Autodesk Inventor part; units mm, degrees
(part 2 of 2)
  line L870 (14, 45.5733) -> (13.8947, 45.8276) construction
  line L871 (13.8947, 45.8276) -> (13.7072, 46.0152) construction
  spline S21 degree 3 poles (13.7072, 46.0152) (13.707012, 46.015387) (13.5196, 46.2027) (13.2653, 46.308) (13, 46.308) knots 0.5 0.5 0.5 0.5 0.50000001 1 1 1 1
  line L872 (13.7072, 46.0152) -> (13.7072, 46.0152) construction
  line L873 (13.7072, 46.0152) -> (13.5196, 46.2027) construction
  line L874 (13.5196, 46.2027) -> (13.2653, 46.308) construction
  line L875 (13.2653, 46.308) -> (13, 46.308) construction
  line L876 (13, 46.308) -> (11, 46.308)
  spline S22 degree 3 poles (11, 46.308) (10.7348, 46.308) (10.4805, 46.2027) (10.2929, 46.0152) knots 0 0 0 0 0.5 0.5 0.5 0.5
  line L877 (11, 46.308) -> (10.7348, 46.308) construction
  line L878 (10.7348, 46.308) -> (10.4805, 46.2027) construction
  line L879 (10.4805, 46.2027) -> (10.2929, 46.0152) construction
  spline S23 degree 3 poles (10.2929, 46.0152) (10.292713, 46.015012) (10.1054, 45.8276) (10, 45.5733) (10, 45.308) knots 0.5 0.5 0.5 0.5 0.50000001 1 1 1 1
  line L880 (10.2929, 46.0152) -> (10.2929, 46.0152) construction
  line L881 (10.2929, 46.0152) -> (10.1054, 45.8276) construction
  line L882 (10.1054, 45.8276) -> (10, 45.5733) construction
  line L883 (10, 45.5733) -> (10, 45.308) construction
  line L884 (10, 45.308) -> (10, 41.3081)
  line L885 (10, 41.3081) -> (9, 41.3081)
  line L886 (9, 41.3081) -> (9, 39.3081)
  line L887 (7, 39.3081) -> (7, 41.3081)
  line L888 (7, 41.3081) -> (6, 41.3081)
  line L889 (6, 41.3081) -> (6, 45.308)
  spline S24 degree 3 poles (6, 45.308) (6, 45.5733) (5.8947, 45.8276) (5.7072, 46.0152) knots 0 0 0 0 0.5 0.5 0.5 0.5
  line L890 (6, 45.308) -> (6, 45.5733) construction
  line L891 (6, 45.5733) -> (5.8947, 45.8276) construction
  line L892 (5.8947, 45.8276) -> (5.7072, 46.0152) construction
  spline S25 degree 3 poles (5.7072, 46.0152) (5.707012, 46.015387) (5.5196, 46.2027) (5.2653, 46.308) (5, 46.308) knots 0.5 0.5 0.5 0.5 0.50000001 1 1 1 1
  line L893 (5.7072, 46.0152) -> (5.7072, 46.0152) construction
  line L894 (5.7072, 46.0152) -> (5.5196, 46.2027) construction
  line L895 (5.5196, 46.2027) -> (5.2653, 46.308) construction
  line L896 (5.2653, 46.308) -> (5, 46.308) construction
  line L897 (5, 46.308) -> (3, 46.308)
  spline S26 degree 3 poles (3, 46.308) (2.7348, 46.308) (2.4805, 46.2027) (2.2929, 46.0152) knots 0 0 0 0 0.5 0.5 0.5 0.5
  line L898 (3, 46.308) -> (2.7348, 46.308) construction
  line L899 (2.7348, 46.308) -> (2.4805, 46.2027) construction
  line L900 (2.4805, 46.2027) -> (2.2929, 46.0152) construction
  spline S27 degree 3 poles (2.2929, 46.0152) (2.292713, 46.015012) (2.1054, 45.8276) (2, 45.5733) (2, 45.308) knots 0.5 0.5 0.5 0.5 0.50000001 1 1 1 1
  line L901 (2.2929, 46.0152) -> (2.2929, 46.0152) construction
  line L902 (2.2929, 46.0152) -> (2.1054, 45.8276) construction
  line L903 (2.1054, 45.8276) -> (2, 45.5733) construction
  line L904 (2, 45.5733) -> (2, 45.308) construction
  line L905 (2, 45.308) -> (2, 41.3081)
  line L906 (2, 41.3081) -> (1, 41.3081)
  line L907 (1, 41.3081) -> (1, 37.6081)
  line L908 (1, 37.6081) -> (7, 37.6081)
  line L909 (7, 37.6081) -> (7, 39.0081)
  line L910 (7, 39.0081) -> (9, 39.0081)
  line L911 (9, 39.3081) -> (7, 39.3081)
  line L912 (61.6606, 20.3061) -> (65.6606, 20.3061)
  line L913 (65.6606, 20.3061) -> (65.6606, 23.3061)
  line L914 (65.6606, 23.3061) -> (61.6606, 23.3061)
  line L915 (61.6606, 23.3061) -> (61.6606, 20.3061)
  line L916 (7.1396, 50.4111) -> (11.1396, 50.4111)
  line L917 (11.1396, 50.4111) -> (11.1396, 53.4111)
  line L918 (11.1396, 53.4111) -> (7.1396, 53.4111)
  line L919 (7.1396, 53.4111) -> (7.1396, 50.4111)
  line L920 (7.1396, 57.4111) -> (11.1396, 57.4111)
  line L921 (11.1396, 57.4111) -> (11.1396, 60.4111)
  line L922 (11.1396, 60.4111) -> (7.1396, 60.4111)
  line L923 (7.1396, 60.4111) -> (7.1396, 57.4111)
  line L924 (173.9998, 64.6598) -> (168.9998, 64.6598)
  line L925 (168.9998, 64.6598) -> (168.9998, 67.6598)
  line L926 (168.9998, 67.6598) -> (173.9998, 67.6598)
  line L927 (173.9998, 67.6598) -> (173.9998, 64.6598)
  line L928 (173.9998, 5.9564) -> (168.9998, 5.9564)
  line L929 (168.9998, 5.9564) -> (168.9998, 2.9564)
  line L930 (168.9998, 2.9564) -> (173.9998, 2.9564)
  line L931 (173.9998, 2.9564) -> (173.9998, 5.9564)
  line L932 (7.1836, 64.6598) -> (12.1836, 64.6598)
  line L933 (12.1836, 64.6598) -> (12.1836, 67.6598)
  line L934 (12.1836, 67.6598) -> (7.1836, 67.6598)
  line L935 (7.1836, 67.6598) -> (7.1836, 64.6598)
  spline S28 degree 3 poles (16.2657, 59.4698) (16.2657, 60.2982) (15.5941, 60.9698) (14.7657, 60.9698) knots 0 0 0 0 1 1 1 1
  line L936 (16.2657, 59.4698) -> (16.2657, 60.2982) construction
  line L937 (16.2657, 60.2982) -> (15.5941, 60.9698) construction
  line L938 (15.5941, 60.9698) -> (14.7657, 60.9698) construction
  line L939 (14.7657, 60.9698) -> (14.7657, 60.9698) construction
  line L940 (14.7657, 60.9698) -> (13.9372, 60.9698) construction
  line L941 (13.9372, 60.9698) -> (13.2657, 60.2982) construction
  line L942 (13.2657, 60.2982) -> (13.2657, 59.4698) construction
  line L943 (13.2657, 59.4698) -> (13.2657, 59.4698) construction
  line L944 (13.2657, 59.4698) -> (13.2657, 58.6414) construction
  line L945 (13.2657, 58.6414) -> (13.9372, 57.9698) construction
  line L946 (13.9372, 57.9698) -> (14.7657, 57.9698) construction
  line L947 (14.7657, 57.9698) -> (14.7657, 57.9698) construction
  line L948 (14.7657, 57.9698) -> (15.5941, 57.9698) construction
  line L949 (15.5941, 57.9698) -> (16.2657, 58.6414) construction
  line L950 (16.2657, 58.6414) -> (16.2657, 59.4698) construction
  spline S29 degree 3 poles (16.2657, 11.2099) (16.2657, 12.0383) (15.5941, 12.7099) (14.7657, 12.7099) knots 0 0 0 0 1 1 1 1
  line L951 (16.2657, 11.2099) -> (16.2657, 12.0383) construction
  line L952 (16.2657, 12.0383) -> (15.5941, 12.7099) construction
  line L953 (15.5941, 12.7099) -> (14.7657, 12.7099) construction
  line L954 (14.7657, 12.7099) -> (14.7657, 12.7099) construction
  line L955 (14.7657, 12.7099) -> (13.9372, 12.7099) construction
  line L956 (13.9372, 12.7099) -> (13.2657, 12.0383) construction
  line L957 (13.2657, 12.0383) -> (13.2657, 11.2099) construction
  line L958 (13.2657, 11.2099) -> (13.2657, 11.2099) construction
  line L959 (13.2657, 11.2099) -> (13.2657, 10.3815) construction
  line L960 (13.2657, 10.3815) -> (13.9372, 9.7099) construction
  line L961 (13.9372, 9.7099) -> (14.7657, 9.7099) construction
  line L962 (14.7657, 9.7099) -> (14.7657, 9.7099) construction
  line L963 (14.7657, 9.7099) -> (15.5941, 9.7099) construction
  line L964 (15.5941, 9.7099) -> (16.2657, 10.3815) construction
  line L965 (16.2657, 10.3815) -> (16.2657, 11.2099) construction
  spline S30 degree 3 poles (82.3057, 14.3849) (82.3057, 15.2133) (81.6341, 15.8849) (80.8057, 15.8849) knots 0 0 0 0 1 1 1 1
  line L966 (82.3057, 14.3849) -> (82.3057, 15.2133) construction
  line L967 (82.3057, 15.2133) -> (81.6341, 15.8849) construction
  line L968 (81.6341, 15.8849) -> (80.8057, 15.8849) construction
  line L969 (80.8057, 15.8849) -> (80.8057, 15.8849) construction
  line L970 (80.8057, 15.8849) -> (79.9772, 15.8849) construction
  line L971 (79.9772, 15.8849) -> (79.3057, 15.2133) construction
  line L972 (79.3057, 15.2133) -> (79.3057, 14.3849) construction
  line L973 (79.3057, 14.3849) -> (79.3057, 14.3849) construction
  line L974 (79.3057, 14.3849) -> (79.3057, 13.5565) construction
  line L975 (79.3057, 13.5565) -> (79.9772, 12.8849) construction
  line L976 (79.9772, 12.8849) -> (80.8057, 12.8849) construction
  line L977 (80.8057, 12.8849) -> (80.8057, 12.8849) construction
  line L978 (80.8057, 12.8849) -> (81.6341, 12.8849) construction
  line L979 (81.6341, 12.8849) -> (82.3057, 13.5565) construction
  line L980 (82.3057, 13.5565) -> (82.3057, 14.3849) construction
  line L981 (0, 13.7411) -> (0, 2.9565)
  line L982 (0, 2.9564) -> (0.0018, 2.854)
  line L983 (0.0018, 2.854) -> (0.007, 2.7517)
  line L984 (0.007, 2.7517) -> (0.0158, 2.6496)
  line L985 (0.0158, 2.6496) -> (0.028, 2.5479)
  line L986 (0.028, 2.5479) -> (0.0437, 2.4467)
  line L987 (0.0437, 2.4467) -> (0.0628, 2.346)
  line L988 (0.0628, 2.346) -> (0.0853, 2.2461)
  line L989 (0.0853, 2.2461) -> (0.1113, 2.147)
  line L990 (0.1113, 2.147) -> (0.1406, 2.0489)
  line L991 (0.1406, 2.0489) -> (0.1733, 1.9518)
  line L992 (0.1733, 1.9518) -> (0.2092, 1.8558)
  line L993 (0.2092, 1.8558) -> (0.2484, 1.7612)
  line L994 (0.2484, 1.7612) -> (0.2908, 1.6679)
  line L995 (0.2908, 1.6679) -> (0.3364, 1.5762)
  line L996 (0.3364, 1.5762) -> (0.3851, 1.4861)
  line L997 (0.3851, 1.4861) -> (0.4368, 1.3976)
  line L998 (0.4368, 1.3976) -> (0.4915, 1.311)
  line L999 (0.4915, 1.311) -> (0.5491, 1.2264)
  line L1000 (0.5491, 1.2264) -> (0.6096, 1.1437)
  line L1001 (0.6096, 1.1437) -> (0.6729, 1.0631)
  line L1002 (0.6729, 1.0631) -> (0.7389, 0.9848)
  line L1003 (0.7389, 0.9848) -> (0.8075, 0.9087)
  line L1004 (0.8075, 0.9087) -> (0.8787, 0.8351)
  line L1005 (0.8787, 0.8351) -> (0.9524, 0.7639)
  line L1006 (0.9524, 0.7639) -> (1.0284, 0.6953)
  line L1007 (1.0284, 0.6953) -> (1.1068, 0.6293)
  line L1008 (1.1068, 0.6293) -> (1.1873, 0.566)
  line L1009 (1.1873, 0.566) -> (1.27, 0.5055)
  line L1010 (1.27, 0.5055) -> (1.3547, 0.4479)
  line L1011 (1.3547, 0.4479) -> (1.4413, 0.3931)
  line L1012 (1.4413, 0.3931) -> (1.5297, 0.3414)
  line L1013 (1.5297, 0.3414) -> (1.6199, 0.2927)
  line L1014 (1.6199, 0.2927) -> (1.7116, 0.2472)
  line L1015 (1.7116, 0.2472) -> (1.8048, 0.2048)
  line L1016 (1.8048, 0.2048) -> (1.8995, 0.1656)
  line L1017 (1.8995, 0.1656) -> (1.9954, 0.1296)
  line L1018 (1.9954, 0.1296) -> (2.0925, 0.097)
  line L1019 (2.0925, 0.097) -> (2.1907, 0.0676)
  line L1020 (2.1907, 0.0676) -> (2.2898, 0.0417)
  line L1021 (2.2898, 0.0417) -> (2.3897, 0.0191)
  line L1022 (2.3897, 0.0191) -> (2.4903, 0)
  line L1023 (2.4903, 0) -> (2.5916, -0.0157)
  line L1024 (2.5916, -0.0157) -> (2.6933, -0.0279)
  line L1025 (2.6933, -0.0279) -> (2.7953, -0.0366)
  line L1026 (2.7953, -0.0366) -> (2.8976, -0.0419)
  line L1027 (2.8976, -0.0419) -> (3, -0.0436)
  line L1028 (3, -0.0436) -> (84, -0.0436)
  line L1029 (84, -0.0436) -> (84.1025, -0.0419)
  line L1030 (84.1025, -0.0419) -> (84.2048, -0.0366)
  line L1031 (84.2048, -0.0366) -> (84.3068, -0.0279)
  line L1032 (84.3068, -0.0279) -> (84.4085, -0.0157)
  line L1033 (84.4085, -0.0157) -> (84.5098, 0)
  line L1034 (84.5098, 0) -> (84.6104, 0.0191)
  line L1035 (84.6104, 0.0191) -> (84.7103, 0.0417)
  line L1036 (84.7103, 0.0417) -> (84.8094, 0.0676)
  line L1037 (84.8094, 0.0676) -> (84.9076, 0.097)
  line L1038 (84.9076, 0.097) -> (85.0047, 0.1296)
  line L1039 (85.0047, 0.1296) -> (85.1006, 0.1656)
  line L1040 (85.1006, 0.1656) -> (85.1953, 0.2048)
  line L1041 (85.1953, 0.2048) -> (85.2885, 0.2472)
  line L1042 (85.2885, 0.2472) -> (85.3802, 0.2927)
  line L1043 (85.3802, 0.2927) -> (85.4704, 0.3414)
  line L1044 (85.4704, 0.3414) -> (85.5588, 0.3931)
  line L1045 (85.5588, 0.3931) -> (85.6454, 0.4479)
  line L1046 (85.6454, 0.4479) -> (85.7301, 0.5055)
  line L1047 (85.7301, 0.5055) -> (85.8128, 0.566)
  line L1048 (85.8128, 0.566) -> (85.8933, 0.6293)
  line L1049 (85.8933, 0.6293) -> (85.9717, 0.6953)
  line L1050 (85.9717, 0.6953) -> (86.0477, 0.7639)
  line L1051 (86.0477, 0.7639) -> (86.1214, 0.8351)
  line L1052 (86.1214, 0.8351) -> (86.1926, 0.9087)
  line L1053 (86.1926, 0.9087) -> (86.2612, 0.9848)
  line L1054 (86.2612, 0.9848) -> (86.3272, 1.0631)
  line L1055 (86.3272, 1.0631) -> (86.3905, 1.1437)
  line L1056 (86.3905, 1.1437) -> (86.451, 1.2264)
  line L1057 (86.451, 1.2264) -> (86.5086, 1.311)
  line L1058 (86.5086, 1.311) -> (86.5633, 1.3976)
  line L1059 (86.5633, 1.3976) -> (86.615, 1.4861)
  line L1060 (86.615, 1.4861) -> (86.6637, 1.5762)
  line L1061 (86.6637, 1.5762) -> (86.7093, 1.6679)
  line L1062 (86.7093, 1.6679) -> (86.7517, 1.7612)
  line L1063 (86.7517, 1.7612) -> (86.7909, 1.8558)
  line L1064 (86.7909, 1.8558) -> (86.8268, 1.9518)
  line L1065 (86.8268, 1.9518) -> (86.8595, 2.0489)
  line L1066 (86.8595, 2.0489) -> (86.8888, 2.147)
  line L1067 (86.8888, 2.147) -> (86.9148, 2.2461)
  line L1068 (86.9148, 2.2461) -> (86.9373, 2.346)
  line L1069 (86.9373, 2.346) -> (86.9564, 2.4467)
  line L1070 (86.9564, 2.4467) -> (86.9721, 2.5479)
  line L1071 (86.9721, 2.5479) -> (86.9843, 2.6496)
  line L1072 (86.9843, 2.6496) -> (86.9931, 2.7517)
  line L1073 (86.9931, 2.7517) -> (86.9983, 2.854)
  line L1074 (86.9983, 2.854) -> (87, 2.9564)
  line L1075 (87, 2.9564) -> (87, 67.6598)
  line L1076 (87, 67.6598) -> (86.9983, 67.7622)
  line L1077 (86.9983, 67.7622) -> (86.9931, 67.8645)
  line L1078 (86.9931, 67.8645) -> (86.9843, 67.9666)
  line L1079 (86.9843, 67.9666) -> (86.9721, 68.0683)
  line L1080 (86.9721, 68.0683) -> (86.9564, 68.1695)
  line L1081 (86.9564, 68.1695) -> (86.9373, 68.2702)
  line L1082 (86.9373, 68.2702) -> (86.9148, 68.3701)
  line L1083 (86.9148, 68.3701) -> (86.8888, 68.4692)
  line L1084 (86.8888, 68.4692) -> (86.8595, 68.5673)
  line L1085 (86.8595, 68.5673) -> (86.8268, 68.6644)
  line L1086 (86.8268, 68.6644) -> (86.7909, 68.7604)
  line L1087 (86.7909, 68.7604) -> (86.7517, 68.855)
  line L1088 (86.7517, 68.855) -> (86.7093, 68.9483)
  line L1089 (86.7093, 68.9483) -> (86.6637, 69.04)
  line L1090 (86.6637, 69.04) -> (86.615, 69.1301)
  line L1091 (86.615, 69.1301) -> (86.5633, 69.2186)
  line L1092 (86.5633, 69.2186) -> (86.5086, 69.3052)
  line L1093 (86.5086, 69.3052) -> (86.451, 69.3898)
  line L1094 (86.451, 69.3898) -> (86.3905, 69.4725)
  line L1095 (86.3905, 69.4725) -> (86.3272, 69.5531)
  line L1096 (86.3272, 69.5531) -> (86.2612, 69.6314)
  line L1097 (86.2612, 69.6314) -> (86.1926, 69.7075)
  line L1098 (86.1926, 69.7075) -> (86.1214, 69.7811)
  line L1099 (86.1214, 69.7811) -> (86.0477, 69.8523)
  line L1100 (86.0477, 69.8523) -> (85.9717, 69.9209)
  line L1101 (85.9717, 69.9209) -> (85.8933, 69.9869)
  line L1102 (85.8933, 69.9869) -> (85.8128, 70.0502)
  line L1103 (85.8128, 70.0502) -> (85.7301, 70.1107)
  line L1104 (85.7301, 70.1107) -> (85.6454, 70.1683)
  line L1105 (85.6454, 70.1683) -> (85.5588, 70.2231)
  line L1106 (85.5588, 70.2231) -> (85.4704, 70.2748)
  line L1107 (85.4704, 70.2748) -> (85.3802, 70.3235)
  line L1108 (85.3802, 70.3235) -> (85.2885, 70.369)
  line L1109 (85.2885, 70.369) -> (85.1953, 70.4114)
  line L1110 (85.1953, 70.4114) -> (85.1006, 70.4506)
  line L1111 (85.1006, 70.4506) -> (85.0047, 70.4866)
  line L1112 (85.0047, 70.4866) -> (84.9076, 70.5192)
  line L1113 (84.9076, 70.5192) -> (84.8094, 70.5486)
  line L1114 (84.8094, 70.5486) -> (84.7103, 70.5745)
  line L1115 (84.7103, 70.5745) -> (84.6104, 70.5971)
  line L1116 (84.6104, 70.5971) -> (84.5098, 70.6162)
  line L1117 (84.5098, 70.6162) -> (84.4085, 70.6319)
  line L1118 (84.4085, 70.6319) -> (84.3068, 70.6441)
  line L1119 (84.3068, 70.6441) -> (84.2048, 70.6528)
  line L1120 (84.2048, 70.6528) -> (84.1025, 70.6581)
  line L1121 (84.1025, 70.6581) -> (84, 70.6598)
  line L1122 (84, 70.6598) -> (3, 70.6598)
  line L1123 (3, 70.6598) -> (2.8976, 70.6581)
  line L1124 (2.8976, 70.6581) -> (2.7953, 70.6528)
  line L1125 (2.7953, 70.6528) -> (2.6933, 70.6441)
  line L1126 (2.6933, 70.6441) -> (2.5916, 70.6319)
  line L1127 (2.5916, 70.6319) -> (2.4903, 70.6162)
  line L1128 (2.4903, 70.6162) -> (2.3897, 70.5971)
  line L1129 (2.3897, 70.5971) -> (2.2898, 70.5745)
  line L1130 (2.2898, 70.5745) -> (2.1907, 70.5486)
  line L1131 (2.1907, 70.5486) -> (2.0925, 70.5192)
  line L1132 (2.0925, 70.5192) -> (1.9954, 70.4866)
  line L1133 (1.9954, 70.4866) -> (1.8995, 70.4506)
  line L1134 (1.8995, 70.4506) -> (1.8048, 70.4114)
  line L1135 (1.8048, 70.4114) -> (1.7116, 70.369)
  line L1136 (1.7116, 70.369) -> (1.6199, 70.3235)
  line L1137 (1.6199, 70.3235) -> (1.5297, 70.2748)
  line L1138 (1.5297, 70.2748) -> (1.4413, 70.2231)
  line L1139 (1.4413, 70.2231) -> (1.3547, 70.1683)
  line L1140 (1.3547, 70.1683) -> (1.27, 70.1107)
  line L1141 (1.27, 70.1107) -> (1.1873, 70.0502)
  line L1142 (1.1873, 70.0502) -> (1.1068, 69.9869)
  line L1143 (1.1068, 69.9869) -> (1.0284, 69.9209)
  line L1144 (1.0284, 69.9209) -> (0.9524, 69.8523)
  line L1145 (0.9524, 69.8523) -> (0.8787, 69.7811)
  line L1146 (0.8787, 69.7811) -> (0.8075, 69.7075)
  line L1147 (0.8075, 69.7075) -> (0.7389, 69.6314)
  line L1148 (0.7389, 69.6314) -> (0.6729, 69.5531)
  line L1149 (0.6729, 69.5531) -> (0.6096, 69.4725)
  line L1150 (0.6096, 69.4725) -> (0.5491, 69.3898)
  line L1151 (0.5491, 69.3898) -> (0.4915, 69.3052)
  line L1152 (0.4915, 69.3052) -> (0.4368, 69.2186)
  line L1153 (0.4368, 69.2186) -> (0.3851, 69.1301)
  line L1154 (0.3851, 69.1301) -> (0.3364, 69.04)
  line L1155 (0.3364, 69.04) -> (0.2908, 68.9483)
  line L1156 (0.2908, 68.9483) -> (0.2484, 68.855)
  line L1157 (0.2484, 68.855) -> (0.2092, 68.7604)
  line L1158 (0.2092, 68.7604) -> (0.1733, 68.6644)
  line L1159 (0.1733, 68.6644) -> (0.1406, 68.5673)
  line L1160 (0.1406, 68.5673) -> (0.1113, 68.4692)
  line L1161 (0.1113, 68.4692) -> (0.0853, 68.3701)
  line L1162 (0.0853, 68.3701) -> (0.0628, 68.2702)
  line L1163 (0.0628, 68.2702) -> (0.0437, 68.1695)
  line L1164 (0.0437, 68.1695) -> (0.028, 68.0683)
  line L1165 (0.028, 68.0683) -> (0.0158, 67.9666)
  line L1166 (0.0158, 67.9666) -> (0.007, 67.8645)
  line L1167 (0.007, 67.8645) -> (0.0018, 67.7622)
  line L1168 (0.0018, 67.7622) -> (0, 67.6598)
  line L1169 (0, 67.6598) -> (0, 48.3081)
  line L1170 (97.1834, 5.9564) -> (102.1834, 5.9564)
  line L1171 (102.1834, 5.9564) -> (102.1834, 2.9564)
  line L1172 (102.1834, 2.9564) -> (97.1834, 2.9564)
  line L1173 (97.1834, 2.9564) -> (97.1834, 5.9564)
  line L1174 (176.9998, 2.9564) -> (176.9998, 67.6598)
  line L1175 (176.9998, 67.6598) -> (176.9981, 67.7622)
  line L1176 (176.9981, 67.7622) -> (176.9929, 67.8645)
  line L1177 (176.9929, 67.8645) -> (176.9841, 67.9666)
  line L1178 (176.9841, 67.9666) -> (176.9719, 68.0683)
  line L1179 (176.9719, 68.0683) -> (176.9562, 68.1695)
  line L1180 (176.9562, 68.1695) -> (176.9371, 68.2702)
  line L1181 (176.9371, 68.2702) -> (176.9146, 68.3701)
  line L1182 (176.9146, 68.3701) -> (176.8886, 68.4692)
  line L1183 (176.8886, 68.4692) -> (176.8593, 68.5673)
  line L1184 (176.8593, 68.5673) -> (176.8266, 68.6644)
  line L1185 (176.8266, 68.6644) -> (176.7907, 68.7604)
  line L1186 (176.7907, 68.7604) -> (176.7515, 68.855)
  line L1187 (176.7515, 68.855) -> (176.7091, 68.9483)
  line L1188 (176.7091, 68.9483) -> (176.6635, 69.04)
  line L1189 (176.6635, 69.04) -> (176.6148, 69.1301)
  line L1190 (176.6148, 69.1301) -> (176.5631, 69.2186)
  line L1191 (176.5631, 69.2186) -> (176.5084, 69.3052)
  line L1192 (176.5084, 69.3052) -> (176.4508, 69.3898)
  line L1193 (176.4508, 69.3898) -> (176.3903, 69.4725)
  line L1194 (176.3903, 69.4725) -> (176.327, 69.5531)
  line L1195 (176.327, 69.5531) -> (176.261, 69.6314)
  line L1196 (176.261, 69.6314) -> (176.1924, 69.7075)
  line L1197 (176.1924, 69.7075) -> (176.1212, 69.7811)
  line L1198 (176.1212, 69.7811) -> (176.0475, 69.8523)
  line L1199 (176.0475, 69.8523) -> (175.9715, 69.9209)
  line L1200 (175.9715, 69.9209) -> (175.8931, 69.9869)
  line L1201 (175.8931, 69.9869) -> (175.8126, 70.0502)
  line L1202 (175.8126, 70.0502) -> (175.7299, 70.1107)
  line L1203 (175.7299, 70.1107) -> (175.6452, 70.1683)
  line L1204 (175.6452, 70.1683) -> (175.5586, 70.2231)
  line L1205 (175.5586, 70.2231) -> (175.4702, 70.2748)
  line L1206 (175.4702, 70.2748) -> (175.38, 70.3235)
  line L1207 (175.38, 70.3235) -> (175.2883, 70.369)
  line L1208 (175.2883, 70.369) -> (175.1951, 70.4114)
  line L1209 (175.1951, 70.4114) -> (175.1004, 70.4506)
  line L1210 (175.1004, 70.4506) -> (175.0045, 70.4866)
  line L1211 (175.0045, 70.4866) -> (174.9074, 70.5192)
  line L1212 (174.9074, 70.5192) -> (174.8092, 70.5486)
  line L1213 (174.8092, 70.5486) -> (174.7101, 70.5745)
  line L1214 (174.7101, 70.5745) -> (174.6102, 70.5971)
  line L1215 (174.6102, 70.5971) -> (174.5096, 70.6162)
  line L1216 (174.5096, 70.6162) -> (174.4083, 70.6319)
  line L1217 (174.4083, 70.6319) -> (174.3066, 70.6441)
  line L1218 (174.3066, 70.6441) -> (174.2046, 70.6528)
  line L1219 (174.2046, 70.6528) -> (174.1023, 70.6581)
  line L1220 (174.1023, 70.6581) -> (173.9998, 70.6598)
  line L1221 (173.9998, 70.6598) -> (92.9999, 70.6598)
  line L1222 (92.9999, 70.6598) -> (92.8975, 70.6581)
  line L1223 (92.8975, 70.6581) -> (92.7952, 70.6528)
  line L1224 (92.7952, 70.6528) -> (92.6932, 70.6441)
  line L1225 (92.6932, 70.6441) -> (92.5915, 70.6319)
  line L1226 (92.5915, 70.6319) -> (92.4902, 70.6162)
  line L1227 (92.4902, 70.6162) -> (92.3896, 70.5971)
  line L1228 (92.3896, 70.5971) -> (92.2897, 70.5745)
  line L1229 (92.2897, 70.5745) -> (92.1906, 70.5486)
  line L1230 (92.1906, 70.5486) -> (92.0924, 70.5192)
  line L1231 (92.0924, 70.5192) -> (91.9953, 70.4866)
  line L1232 (91.9953, 70.4866) -> (91.8994, 70.4506)
  line L1233 (91.8994, 70.4506) -> (91.8047, 70.4114)
  line L1234 (91.8047, 70.4114) -> (91.7115, 70.369)
  line L1235 (91.7115, 70.369) -> (91.6198, 70.3235)
  line L1236 (91.6198, 70.3235) -> (91.5296, 70.2748)
  line L1237 (91.5296, 70.2748) -> (91.4412, 70.2231)
  line L1238 (91.4412, 70.2231) -> (91.3546, 70.1683)
  line L1239 (91.3546, 70.1683) -> (91.2699, 70.1107)
  line L1240 (91.2699, 70.1107) -> (91.1872, 70.0502)
  line L1241 (91.1872, 70.0502) -> (91.1067, 69.9869)
  line L1242 (91.1067, 69.9869) -> (91.0283, 69.9209)
  line L1243 (91.0283, 69.9209) -> (90.9523, 69.8523)
  line L1244 (90.9523, 69.8523) -> (90.8786, 69.7811)
  line L1245 (90.8786, 69.7811) -> (90.8074, 69.7075)
  line L1246 (90.8074, 69.7075) -> (90.7388, 69.6314)
  line L1247 (90.7388, 69.6314) -> (90.6728, 69.5531)
  line L1248 (90.6728, 69.5531) -> (90.6095, 69.4725)
  line L1249 (90.6095, 69.4725) -> (90.549, 69.3898)
  line L1250 (90.549, 69.3898) -> (90.4914, 69.3052)
  line L1251 (90.4914, 69.3052) -> (90.4367, 69.2186)
  line L1252 (90.4367, 69.2186) -> (90.385, 69.1301)
  line L1253 (90.385, 69.1301) -> (90.3363, 69.04)
  line L1254 (90.3363, 69.04) -> (90.2907, 68.9483)
  line L1255 (90.2907, 68.9483) -> (90.2483, 68.855)
  line L1256 (90.2483, 68.855) -> (90.2091, 68.7604)
  line L1257 (90.2091, 68.7604) -> (90.1732, 68.6644)
  line L1258 (90.1732, 68.6644) -> (90.1405, 68.5673)
  line L1259 (90.1405, 68.5673) -> (90.1112, 68.4692)
  line L1260 (90.1112, 68.4692) -> (90.0852, 68.3701)
  line L1261 (90.0852, 68.3701) -> (90.0627, 68.2702)
  line L1262 (90.0627, 68.2702) -> (90.0436, 68.1695)
  line L1263 (90.0436, 68.1695) -> (90.0279, 68.0683)
  line L1264 (90.0279, 68.0683) -> (90.0157, 67.9666)
  line L1265 (90.0157, 67.9666) -> (90.0069, 67.8645)
  line L1266 (90.0069, 67.8645) -> (90.0017, 67.7622)
  line L1267 (90.0017, 67.7622) -> (89.9999, 67.6598)
  line L1268 (89.9999, 67.6598) -> (89.9999, 2.9564)
  line L1269 (89.9999, 2.9564) -> (90.0017, 2.854)
  line L1270 (90.0017, 2.854) -> (90.0069, 2.7517)
  line L1271 (90.0069, 2.7517) -> (90.0157, 2.6496)
  line L1272 (90.0157, 2.6496) -> (90.0279, 2.5479)
  line L1273 (90.0279, 2.5479) -> (90.0436, 2.4467)
  line L1274 (90.0436, 2.4467) -> (90.0627, 2.346)
  line L1275 (90.0627, 2.346) -> (90.0852, 2.2461)
  line L1276 (90.0852, 2.2461) -> (90.1112, 2.147)
  line L1277 (90.1112, 2.147) -> (90.1405, 2.0489)
  line L1278 (90.1405, 2.0489) -> (90.1732, 1.9518)
  line L1279 (90.1732, 1.9518) -> (90.2091, 1.8558)
  line L1280 (90.2091, 1.8558) -> (90.2483, 1.7612)
  line L1281 (90.2483, 1.7612) -> (90.2907, 1.6679)
  line L1282 (90.2907, 1.6679) -> (90.3363, 1.5762)
  line L1283 (90.3363, 1.5762) -> (90.385, 1.4861)
  line L1284 (90.385, 1.4861) -> (90.4367, 1.3976)
  line L1285 (90.4367, 1.3976) -> (90.4914, 1.311)
  line L1286 (90.4914, 1.311) -> (90.549, 1.2264)
  line L1287 (90.549, 1.2264) -> (90.6095, 1.1437)
  line L1288 (90.6095, 1.1437) -> (90.6728, 1.0631)
  line L1289 (90.6728, 1.0631) -> (90.7388, 0.9848)
  line L1290 (90.7388, 0.9848) -> (90.8074, 0.9087)
  line L1291 (90.8074, 0.9087) -> (90.8786, 0.8351)
  line L1292 (90.8786, 0.8351) -> (90.9523, 0.7639)
  line L1293 (90.9523, 0.7639) -> (91.0283, 0.6953)
  line L1294 (91.0283, 0.6953) -> (91.1067, 0.6293)
  line L1295 (91.1067, 0.6293) -> (91.1872, 0.566)
  line L1296 (91.1872, 0.566) -> (91.2699, 0.5055)
  line L1297 (91.2699, 0.5055) -> (91.3546, 0.4479)
  line L1298 (91.3546, 0.4479) -> (91.4412, 0.3931)
  line L1299 (91.4412, 0.3931) -> (91.5296, 0.3414)
  line L1300 (91.5296, 0.3414) -> (91.6198, 0.2927)
  line L1301 (91.6198, 0.2927) -> (91.7115, 0.2472)
  line L1302 (91.7115, 0.2472) -> (91.8047, 0.2048)
  line L1303 (91.8047, 0.2048) -> (91.8994, 0.1656)
  line L1304 (91.8994, 0.1656) -> (91.9953, 0.1296)
  line L1305 (91.9953, 0.1296) -> (92.0924, 0.097)
  line L1306 (92.0924, 0.097) -> (92.1906, 0.0676)
  line L1307 (92.1906, 0.0676) -> (92.2897, 0.0417)
  line L1308 (92.2897, 0.0417) -> (92.3896, 0.0191)
  line L1309 (92.3896, 0.0191) -> (92.4902, 0)
  line L1310 (92.4902, 0) -> (92.5915, -0.0157)
  line L1311 (92.5915, -0.0157) -> (92.6932, -0.0279)
  line L1312 (92.6932, -0.0279) -> (92.7952, -0.0366)
  line L1313 (92.7952, -0.0366) -> (92.8975, -0.0419)
  line L1314 (92.8975, -0.0419) -> (92.9999, -0.0436)
  line L1315 (92.9999, -0.0436) -> (173.9998, -0.0436)
  line L1316 (173.9998, -0.0436) -> (174.1023, -0.0419)
  line L1317 (174.1023, -0.0419) -> (174.2046, -0.0366)
  line L1318 (174.2046, -0.0366) -> (174.3066, -0.0279)
  line L1319 (174.3066, -0.0279) -> (174.4083, -0.0157)
  line L1320 (174.4083, -0.0157) -> (174.5096, 0)
  line L1321 (174.5096, 0) -> (174.6102, 0.0191)
  line L1322 (174.6102, 0.0191) -> (174.7101, 0.0417)
  line L1323 (174.7101, 0.0417) -> (174.8092, 0.0676)
  line L1324 (174.8092, 0.0676) -> (174.9074, 0.097)
  line L1325 (174.9074, 0.097) -> (175.0045, 0.1296)
  line L1326 (175.0045, 0.1296) -> (175.1004, 0.1656)
  line L1327 (175.1004, 0.1656) -> (175.1951, 0.2048)
  line L1328 (175.1951, 0.2048) -> (175.2883, 0.2472)
  line L1329 (175.2883, 0.2472) -> (175.38, 0.2927)
  line L1330 (175.38, 0.2927) -> (175.4702, 0.3414)
  line L1331 (175.4702, 0.3414) -> (175.5586, 0.3931)
  line L1332 (175.5586, 0.3931) -> (175.6452, 0.4479)
  line L1333 (175.6452, 0.4479) -> (175.7299, 0.5055)
  line L1334 (175.7299, 0.5055) -> (175.8126, 0.566)
  line L1335 (175.8126, 0.566) -> (175.8931, 0.6293)
  line L1336 (175.8931, 0.6293) -> (175.9715, 0.6953)
  line L1337 (175.9715, 0.6953) -> (176.0475, 0.7639)
  line L1338 (176.0475, 0.7639) -> (176.1212, 0.8351)
  line L1339 (176.1212, 0.8351) -> (176.1924, 0.9087)
  line L1340 (176.1924, 0.9087) -> (176.261, 0.9848)
  line L1341 (176.261, 0.9848) -> (176.327, 1.0631)
  line L1342 (176.327, 1.0631) -> (176.3903, 1.1437)
  line L1343 (176.3903, 1.1437) -> (176.4508, 1.2264)
  line L1344 (176.4508, 1.2264) -> (176.5084, 1.311)
  line L1345 (176.5084, 1.311) -> (176.5631, 1.3976)
  line L1346 (176.5631, 1.3976) -> (176.6148, 1.4861)
  line L1347 (176.6148, 1.4861) -> (176.6635, 1.5762)
  line L1348 (176.6635, 1.5762) -> (176.7091, 1.6679)
  line L1349 (176.7091, 1.6679) -> (176.7515, 1.7612)
  line L1350 (176.7515, 1.7612) -> (176.7907, 1.8558)
  line L1351 (176.7907, 1.8558) -> (176.8266, 1.9518)
  line L1352 (176.8266, 1.9518) -> (176.8593, 2.0489)
  line L1353 (176.8593, 2.0489) -> (176.8886, 2.147)
  line L1354 (176.8886, 2.147) -> (176.9146, 2.2461)
  line L1355 (176.9146, 2.2461) -> (176.9371, 2.346)
  line L1356 (176.9371, 2.346) -> (176.9562, 2.4467)
  line L1357 (176.9562, 2.4467) -> (176.9719, 2.5479)
  line L1358 (176.9719, 2.5479) -> (176.9841, 2.6496)
  line L1359 (176.9841, 2.6496) -> (176.9929, 2.7517)
  line L1360 (176.9929, 2.7517) -> (176.9981, 2.854)
  line L1361 (176.9981, 2.854) -> (176.9998, 2.9564)
  spline S31 degree 3 poles (172.3055, 14.3849) (172.3055, 15.2133) (171.6339, 15.8849) (170.8055, 15.8849) knots 0 0 0 0 1 1 1 1
  line L1362 (172.3055, 14.3849) -> (172.3055, 15.2133) construction
  line L1363 (172.3055, 15.2133) -> (171.6339, 15.8849) construction
  line L1364 (171.6339, 15.8849) -> (170.8055, 15.8849) construction
  line L1365 (170.8055, 15.8849) -> (170.8055, 15.8849) construction
  line L1366 (170.8055, 15.8849) -> (169.977, 15.8849) construction
  line L1367 (169.977, 15.8849) -> (169.3055, 15.2133) construction
  line L1368 (169.3055, 15.2133) -> (169.3055, 14.3849) construction
  line L1369 (169.3055, 14.3849) -> (169.3055, 14.3849) construction
  line L1370 (169.3055, 14.3849) -> (169.3055, 13.5565) construction
  line L1371 (169.3055, 13.5565) -> (169.977, 12.8849) construction
  line L1372 (169.977, 12.8849) -> (170.8055, 12.8849) construction
  line L1373 (170.8055, 12.8849) -> (170.8055, 12.8849) construction
  line L1374 (170.8055, 12.8849) -> (171.6339, 12.8849) construction
  line L1375 (171.6339, 12.8849) -> (172.3055, 13.5565) construction
  line L1376 (172.3055, 13.5565) -> (172.3055, 14.3849) construction
  spline S32 degree 3 poles (106.2655, 11.2099) (106.2655, 12.0383) (105.5939, 12.7099) (104.7655, 12.7099) knots 0 0 0 0 1 1 1 1
  line L1377 (106.2655, 11.2099) -> (106.2655, 12.0383) construction
  line L1378 (106.2655, 12.0383) -> (105.5939, 12.7099) construction
  line L1379 (105.5939, 12.7099) -> (104.7655, 12.7099) construction
  line L1380 (104.7655, 12.7099) -> (104.7655, 12.7099) construction
  line L1381 (104.7655, 12.7099) -> (103.937, 12.7099) construction
  line L1382 (103.937, 12.7099) -> (103.2655, 12.0383) construction
  line L1383 (103.2655, 12.0383) -> (103.2655, 11.2099) construction
  line L1384 (103.2655, 11.2099) -> (103.2655, 11.2099) construction
  line L1385 (103.2655, 11.2099) -> (103.2655, 10.3815) construction
  line L1386 (103.2655, 10.3815) -> (103.937, 9.7099) construction
  line L1387 (103.937, 9.7099) -> (104.7655, 9.7099) construction
  line L1388 (104.7655, 9.7099) -> (104.7655, 9.7099) construction
  line L1389 (104.7655, 9.7099) -> (105.5939, 9.7099) construction
  line L1390 (105.5939, 9.7099) -> (106.2655, 10.3815) construction
  line L1391 (106.2655, 10.3815) -> (106.2655, 11.2099) construction
  spline S33 degree 3 poles (106.2655, 59.4698) (106.2655, 60.2982) (105.5939, 60.9698) (104.7655, 60.9698) knots 0 0 0 0 1 1 1 1
  line L1392 (106.2655, 59.4698) -> (106.2655, 60.2982) construction
  line L1393 (106.2655, 60.2982) -> (105.5939, 60.9698) construction
  line L1394 (105.5939, 60.9698) -> (104.7655, 60.9698) construction
  line L1395 (104.7655, 60.9698) -> (104.7655, 60.9698) construction
  line L1396 (104.7655, 60.9698) -> (103.937, 60.9698) construction
  line L1397 (103.937, 60.9698) -> (103.2655, 60.2982) construction
  line L1398 (103.2655, 60.2982) -> (103.2655, 59.4698) construction
  line L1399 (103.2655, 59.4698) -> (103.2655, 59.4698) construction
  line L1400 (103.2655, 59.4698) -> (103.2655, 58.6414) construction
  line L1401 (103.2655, 58.6414) -> (103.937, 57.9698) construction
  line L1402 (103.937, 57.9698) -> (104.7655, 57.9698) construction
  line L1403 (104.7655, 57.9698) -> (104.7655, 57.9698) construction
  line L1404 (104.7655, 57.9698) -> (105.5939, 57.9698) construction
  line L1405 (105.5939, 57.9698) -> (106.2655, 58.6414) construction
  line L1406 (106.2655, 58.6414) -> (106.2655, 59.4698) construction
  line L1407 (97.1834, 64.6598) -> (102.1834, 64.6598)
  line L1408 (102.1834, 64.6598) -> (102.1834, 67.6598)
  line L1409 (102.1834, 67.6598) -> (97.1834, 67.6598)
  line L1410 (97.1834, 67.6598) -> (97.1834, 64.6598)
  line L1411 (57, 14.0208) -> (57, 17.3081)
  line L1412 (57, 17.3081) -> (41, 17.3081)
  line L1413 (41, 17.3081) -> (41, 14.0208)
  line L1414 (57, 14.0208) -> (77.5335, 14.0208)
  line L1415 (77.5335, 14.0208) -> (77.5335, 8.3081)
  line L1416 (77.5335, 8.3081) -> (18, 8.3081)
  line L1417 (18, 8.3081) -> (18, 14.0208)
  line L1418 (18, 14.0208) -> (41, 14.0208)
  line L1419 (84, 64.6598) -> (79, 64.6598)
  line L1420 (79, 64.6598) -> (79, 67.6598)
  line L1421 (79, 67.6598) -> (84, 67.6598)
  line L1422 (84, 67.6598) -> (84, 64.6598)
  line L1423 (84, 5.9564) -> (79, 5.9564)
  line L1424 (79, 5.9564) -> (79, 2.9564)
  line L1425 (79, 2.9564) -> (84, 2.9564)
  line L1426 (84, 2.9564) -> (84, 5.9564)
  line L1427 (0, 32.2411) -> (0, 29.8082)
  line L1428 (0, 13.7411) -> (16.5081, 13.7411)
  line L1429 (16.5081, 13.7411) -> (16.5081, 29.8081)
  line L1430 (16.5081, 29.8081) -> (0, 29.8081)
  line L1431 (0, 32.2411) -> (16.5081, 32.2411)
  line L1432 (16.5081, 32.2411) -> (16.5081, 48.308)
  line L1433 (16.5081, 48.308) -> (0, 48.308)
  line L1434 (7.1836, 5.9564) -> (12.1836, 5.9564)
  line L1435 (12.1836, 5.9564) -> (12.1836, 2.9564)
  line L1436 (12.1836, 2.9564) -> (7.1836, 2.9564)
  line L1437 (7.1836, 2.9564) -> (7.1836, 5.9564)
  line L1438 (18, 56.5954) -> (77.5335, 56.5954)
  line L1439 (77.5335, 56.5954) -> (77.5335, 62.308)
  line L1440 (77.5335, 62.308) -> (18, 62.308)
  line L1441 (18, 62.308) -> (18, 56.5954)
  line L1442 (79.00054, 75.9421) -> (12.18414, 75.9421)
  line L1443 (79, 88.5421) -> (12.1836, 88.5421)
  line L1444 (84, 88.5415) -> (87.0001, 88.5415)
  line L1445 (84.0001, 75.9421) -> (87.0001, 75.9421)
  line L1446 (84.0001, 75.9421) -> (84.0001, 72.9421)
  line L1447 (84.0001, 75.9421) -> (88.247672, 75.9421) construction
  line L1448 (79.00054, 75.9421) -> (79.00054, 72.9421)
  line L1449 (84, 88.5415) -> (84, 91.5415)
  line L1450 (84, 88.5415) -> (87.0001, 88.5415) construction
  line L1451 (79, 88.5421) -> (79, 91.5415)
  line L1452 (79, 88.5421) -> (84.935098, 88.5421) construction
  line L1453 (7.18414, 75.9421) -> (0.0001, 75.9421)
  line L1454 (7.18414, 75.9421) -> (7.18414, 72.9421)
  line L1455 (12.18414, 75.9421) -> (12.18414, 72.9421)
  line L1456 (7.1836, 88.5421) -> (0.0001, 88.5421)
  line L1457 (7.1836, 88.5421) -> (16.500145, 88.5421) construction
  line L1458 (7.1836, 88.5421) -> (7.1836, 91.5421)
  line L1459 (7.1836, 88.5421) -> (12.115341, 88.5421) construction
  line L1460 (12.1836, 88.5421) -> (12.1836, 91.5421)
  line L1461 (12.1836, 88.5421) -> (18.118698, 88.5421) construction
  line L1462 (8.1836, 91.5421) -> (12.0471, 91.5421) construction
  line L1463 (11.18414, 72.9421) -> (12.43139, 72.9421) construction
  line L1464 (8.1836, 72.9421) -> (10.8476, 72.9421) construction
  line L1465 (12.1836, 91.5421) -> (7.1836, 91.5421)
  line L1466 (12.18414, 72.9421) -> (7.18414, 72.9421)
  line L1467 (0.0001, 88.5421) -> (0.0001, 75.9421)
  line L1468 (83.0002, 72.9421) -> (85.149803, 72.9421) construction
  line L1469 (80, 72.9421) -> (82.529083, 72.9421) construction
  line L1470 (79.9659, 91.5415) -> (82.172325, 91.5415) construction
  line L1471 (79, 91.5415) -> (84, 91.5415)
  line L1472 (87.0001, 88.5415) -> (87.0001, 75.9421)
  line L1473 (84.0001, 72.9421) -> (79.00054, 72.9421)
  point P0 (0, 0)
  dimension "d0" = 90
  dimension "d1" = 90
  dimension "d2" = 90
  dimension "d3" = 180
  dimension "d4" = 90
  dimension "d6" = 90
  constraints: 2576 end point, 17 horizontal, 2 equal length, 2 perpendicular, 2 point on line, 2 vertical, 102 other
  measures "d0" angle of L1446 L1447
  measures "d1" angle of L1450 L1449
  measures "d2" angle of L1452 L1451
  measures "d3" angle of L1456 L1457
  measures "d4" angle of L1459 L1458
  measures "d6" angle of L1461 L1460
extrude "Extrusion1" add sketch "Sketch1" along normal blind 3 contours S11 L812 L811 L810 L809 L808 L807 L806 L805 L804 L803 L802 L801 L800 L799 L798 L797 L796 L795 L794 L793 L792 L791 L790 L789 L788 L787 L786 L785 L784 L783 L782 L781 L780 L779 L778 L777 L776 L775 L774 L773 L772 L771 L770 L769 L768 L767 L766 L765 L764 L763 L762 L761 L760 L759 L758 L757 L756 L755 L754 L753 L752 L751 L750 L749 L748 L747 L746 L745 L744 L743 L742 L741 L740 L739 L738 L737 L736 L735 L734 L733 L732 L731 L730 L729 L728 L727 L726 L725 L724 L723 L722 L721 L720 L719 L718 L717 L716 L715 L714 L713 L712 L711 L710 L709 L708 L707 L706 L705 L704 L703 L702 L701 L700 L699 L698 L697 L696 L695 L694 L693 L692 L691 L690 L689 L688 L687 L686 L685 L684 L683 L682 L681 L680 L679 L678 L677 L676 L675 L674 L673 L672 L671 L670 L669 L668 L667 L666 L665 L664 L663 L662 L661 L660 L659 L658 L657 L656 L655 L654 L653 L652 L651 L650 L649 L648 L647 L646 L645 L644 L643 L642 L641 L640 L639 L638 L637 L636 L635 L634 L633 L632 L631 L630 L629 L628 L627 L626 L625 L624 L623 L622 L621 L620 S10 S9 L612 S8 S7 L604 L603 L602 L601 L600 L599 L598 L597 L596 L595 L594 L593 L592 L591 L590 L589 L588 L587 L586 L585 L584 L583 L582 L581 L580 L579 L578 L577 L576 L575 L574 L573 L572 L571 L570 L569 L568 L567 L566 L565 L564 L563 L562 L561 L560 L559 L558 L557 L556 L555 L554 L553 L552 L551 L550 L549 L548 L547 L546 L545 L544 L543 L542 L541 L540 L539 L538 L537 L536 L535 L534 L533 L532 L531 L530 L529 L528 L527 L526 L525 L524 L523 L522 L521 L520 L519 L518 L517 L516 L515 L514 L513 L512 L511 L510 L509 L508 L507 L506 L505 L504 L503 L502 L501 L500 L499 L498 L497 L496 L495 L494 L493 L492 L491 L490 L489 L488 L487 L486 L485 L484 L483 L482 L481 L480 L479 L478 L477 L476 L475 L474 L473 L472 L471 L470 L469 L468 L467 L466 L465 L464 L463 L462 L461 L460 L459 L458 L457 L456 L455 L454 L453 L452 L451 L450 L449 L448 L447 L446 L445 L444 L443 L442 L441 L440 L439 L438 L437 L436 L435 L434 L433 L432 L431 L430 L429 L428 L427 L426 L425 L424 L423 L422 L421 L420 L419 L418 L417 L416 L415 L414 L413 L412 S6 L408 | L1472 L1445 S11 | S6 L1444 L1472 | L1446 L1473 L766 L767 L768 L769 L770 L771 L772 L773 L774 L775 L776 L777 L778 L779 L780 L781 L782 L783 L784 L785 L786 L787 L788 L789 L790 L791 L792 L793 L794 L795 L796 L797 L798 L799 L800 L801 L802 L803 L804 L805 L806 L807 L808 L809 | L415 L416 L417 L418 L419 L420 L421 L422 L423 L424 L425 L426 L427 L428 L429 L430 L431 L432 L433 L434 L435 L436 L437 L438 L439 L440 L441 L442 L443 L444 L445 L446 L447 L448 L449 L450 L451 L452 L453 L454 L455 L456 L457 L1471 L1449 | L1473 L1448 L720 L721 L722 L723 L724 L725 L726 L727 L728 L729 L730 L731 L732 L733 L734 L735 L736 L737 L738 L739 L740 L741 L742 L743 L744 L745 L746 L747 L748 L749 L750 L751 L752 L753 L754 L755 L756 L757 L758 L759 L760 L761 L762 | L463 L464 L465 L466 L467 L468 L469 L470 L471 L472 L473 L474 L475 L476 L477 L478 L479 L480 L481 L482 L483 L484 L485 L486 L487 L488 L489 L490 L491 L492 L493 L494 L495 L496 L497 L498 L499 L500 L501 L502 L503 L504 L505 L1451 L1471 | L1455 L1466 L670 L671 L672 L673 L674 L675 L676 L677 L678 L679 L680 L681 L682 L683 L684 L685 L686 L687 L688 L689 L690 L691 L692 L693 L694 L695 L696 L697 L698 L699 L700 L701 L702 L703 L704 L705 L706 L707 L708 L709 L710 L711 L712 L713 | L511 L512 L513 L514 L515 L516 L517 L518 L519 L520 L521 L522 L523 L524 L525 L526 L527 L528 L529 L530 L531 L532 L533 L534 L535 L536 L537 L538 L539 L540 L541 L542 L543 L544 L545 L546 L547 L548 L549 L550 L551 L552 L553 L554 L1465 L1460 | L1466 L1454 L623 L624 L625 L626 L627 L628 L629 L630 L631 L632 L633 L634 L635 L636 L637 L638 L639 L640 L641 L642 L643 L644 L645 L646 L647 L648 L649 L650 L651 L652 L653 L654 L655 L656 L657 L658 L659 L660 L661 L662 L663 L664 L665 L666 | L558 L559 L560 L561 L562 L563 L564 L565 L566 L567 L568 L569 L570 L571 L572 L573 L574 L575 L576 L577 L578 L579 L580 L581 L582 L583 L584 L585 L586 L587 L588 L589 L590 L591 L592 L593 L594 L595 L596 L597 L598 L599 L600 L601 L1458 L1465 | L1453 L1467 S9 S10 | S7 S8 L1467 L1456
fillet "Fillet1" radius 2 12 edges at (-79, 1.5, 91.5415) (-84, 1.5, 91.5415) (-79.0005, 1.5, 72.9421) (-84.0001, 1.5, 72.9421) (-7.1836, 1.5, 91.5421) (-12.1836, 1.5, 91.5421) (-7.1841, 1.5, 72.9421) (-12.1841, 1.5, 72.9421) (-0.0001, 1.5, 88.5421) (-0.0001, 1.5, 75.9421) (-87.0001, 1.5, 75.9421) (-87.0001, 1.5, 88.5415)
body "Solid1"
